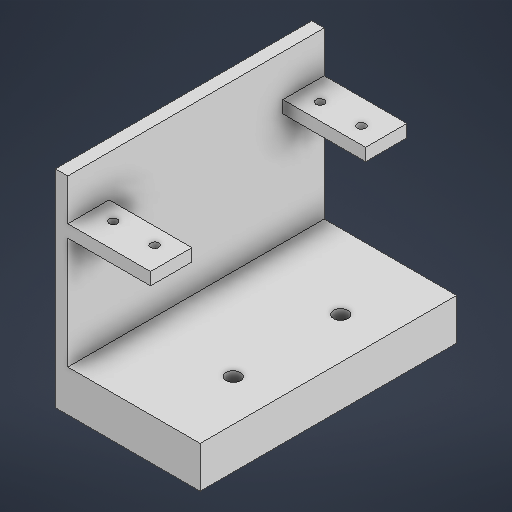
# Autodesk Inventor part: 1.1.2.Mounting1
Saved by Autodesk Inventor 2026.1 (Build 301233020, 233B)
## iProperties
Created: 2025-10-08
Part Number: 1.1.2.Mounting1
Material: Genérico
Document SubType Name: Modeling
Designer: vitos
Density: 1 g/cm^3
Appearance: Valor por defecto
Author: vitos
Autodesk Inventor part; units mm, degrees
ref_plane "YZ Plane" through (0, 0, 0) normal (1, 0, 0) x (0, 1, 0)
ref_plane "XZ Plane" through (0, 0, 0) normal (0, 1, 0) x (-1, 0, 0)
ref_plane "XY Plane" through (0, 0, 0) normal (0, 0, 1) x (1, 0, 0)
sketch "Boceto1" plane through (0, 0, 0) normal (0, 1, 0) x (-1, 0, 0)
  line L0 (0, 0) -> (35, 0)
  line L1 (35, 0) -> (35, -62)
  line L2 (35, -62) -> (0, -62)
  line L3 (0, -62) -> (0, 0)
  line L4 (35, 0) -> (32, 0)
  line L5 (32, 0) -> (32, -62)
  line L6 (32, -62) -> (35, -62)
  line L7 (35, -62) -> (35, 0)
  line L8 (32, 0) -> (12, 0)
  line L9 (12, 0) -> (12, -10)
  line L10 (12, -10) -> (32, -10)
  line L11 (32, -10) -> (32, 0)
  line L12 (32, -62) -> (12, -62)
  line L13 (12, -62) -> (12, -52)
  line L14 (12, -52) -> (32, -52)
  line L15 (32, -52) -> (32, -62)
  circle A0 centre (10, -18) radius 1.75
  circle A1 centre (10, -44) radius 1.75
  circle A2 centre (27, -6) radius 1
  circle A3 centre (17, -6) radius 1
  circle A4 centre (27, -56) radius 1
  circle A5 centre (17, -56) radius 1
  dimension "d0" = 35
  dimension "d1" = 62
  dimension "d2" = 3
  dimension "d3" = 20
  dimension "d4" = 10
  dimension "d5" = 20
  dimension "d6" = 10
  dimension "d7" = 3.5
  dimension "d8" = 3.5
  dimension "d9" = 2
  dimension "d10" = 2
  dimension "d11" = 2
  dimension "d12" = 2
  constraints: 32 end point, 8 parallel, 6 centre point, 4 horizontal, 4 perpendicular, 1 point on line
  measures "d0" distance of L1.end L2.end
  measures "d1" distance of L0.end L1.end
  measures "d2" distance of L6.end L5.end
  measures "d3" distance of L10.end L9.end
  measures "d4" distance of L9.end L8.end
  measures "d5" distance of L13.end L14.end
  measures "d6" distance of L12.end L13.end
  measures "d7" diameter of A0
  measures "d8" diameter of A1
  measures "d9" diameter of A2
  measures "d10" diameter of A3
  measures "d11" diameter of A4
  measures "d12" diameter of A5
extrude "Extrusión1" add sketch "Boceto1" along normal blind 50 contours L0 L1 L2 L5
extrude "Extrusión2" add sketch "Boceto1" along normal blind 10 contours L0 L9 L10 L5 L14 L13 L2 L3 | L0 L5 L10 L9 | L13 L14 L5 L2 | A2 | A3 | A4 | A5
sketch "Boceto2" plane through (-32, 50, 0) normal (1, 0, 0) x (0, 0, -1)
  line L0 (0, -10) -> (10, -10)
  line L1 (10, -10) -> (10, -13)
  line L2 (10, -13) -> (0, -13)
  line L3 (0, -13) -> (0, -10)
  line L4 (62, -50) -> (62, 0) projected
  line L5 (62, -10) -> (52, -10)
  line L6 (52, -10) -> (52, -13)
  line L7 (52, -13) -> (62, -13)
  line L8 (62, -13) -> (62, -10)
  point P0 (0, -50)
  point P1 (62, -13)
  dimension "d17" = 10
  dimension "d18" = 3
  dimension "d19" = 10
  dimension "d20" = 3
  constraints: 16 end point, 4 parallel, 2 horizontal, 2 perpendicular, 1 point on line
  measures "d17" distance of L1.end L2.end
  measures "d18" distance of L0.end L1.end
  measures "d19" distance of L7.end L6.end
  measures "d20" distance of L6.end L5.end
extrude "Extrusión3" add sketch "Boceto2" along normal blind 20
sketch "Boceto3" plane through (-32, 40, 0) normal (0, 1, 0) x (1, 0, 0)
  circle A0 centre (5, 6) radius 1
  circle A1 centre (15, 6) radius 1
  circle A2 centre (5, 56) radius 1
  circle A3 centre (15, 56) radius 1
  point P0 (32, 0)
  dimension "d23" = 2
  dimension "d24" = 2
  dimension "d25" = 2
  dimension "d26" = 2
  constraints: 4 centre point
  measures "d23" diameter of A0
  measures "d24" diameter of A1
  measures "d25" diameter of A2
  measures "d26" diameter of A3
extrude "Extrusión4" cut sketch "Boceto3" against normal blind 3
